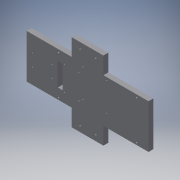
# Autodesk Inventor part: Основная пластина платформы
Saved by Autodesk Inventor 2019.1 (Build 231200000, 200)
## iProperties
Created: 2018-10-15
Part Number: Основная пластина платформы
Material: Типовые
Document SubType Name: Modeling
Designer: Олег
Density: 1 g/cm^3
Appearance: По умолчанию
Author: Олег
Autodesk Inventor part; units mm, degrees
ref_plane "YZ Plane" through (0, 0, 0) normal (1, 0, 0) x (0, 1, 0)
ref_plane "XZ Plane" through (0, 0, 0) normal (0, 1, 0) x (-1, 0, 0)
ref_plane "XY Plane" through (0, 0, 0) normal (0, 0, 1) x (1, 0, 0)
sketch "Эскиз1" plane through (0, 0, 0) normal (0, 0, 1) x (1, 0, 0)
  line L0 (-125, -45) -> (125, -45)
  line L1 (125, -45) -> (125, 45)
  line L2 (125, 45) -> (-125, 45)
  line L3 (-125, 45) -> (-125, -45)
  line L4 (-125, -45) -> (125, 45) construction
  line L5 (125, -45) -> (-125, 45) construction
  line L6 (32.5, -80) -> (-32.5, -80)
  line L7 (-32.5, -80) -> (-32.5, 80)
  line L8 (-32.5, 80) -> (32.5, 80)
  line L9 (32.5, 80) -> (32.5, -80)
  line L10 (32.5, -80) -> (-32.5, 80) construction
  line L11 (-32.5, -80) -> (32.5, 80) construction
  point P0 (0, 0)
  dimension "d0" = 250
  dimension "d1" = 90
  dimension "d2" = 65
  dimension "d3" = 160
  constraints: 24 end point, 4 midpoint, 4 parallel, 2 horizontal, 2 perpendicular
  measures "d0" distance of L2.end L1.end
  measures "d1" distance of L1.end L0.end
  measures "d2" distance of L7.end L8.end
  measures "d3" distance of L6.end L7.end
extrude "Выдавливание1" add sketch "Эскиз1" along normal blind 10
sketch "Эскиз2" plane through (0, 0, 10) normal (0, 0, 1) x (1, 0, 0)
  line L0 (16, 68) -> (-16, 68) construction
  line L1 (-16, 68) -> (-16, 80) construction
  line L2 (-16, 80) -> (16, 80) construction
  line L3 (16, 80) -> (16, 68) construction
  line L4 (16, 68) -> (-16, 80) construction
  line L5 (-16, 68) -> (16, 80) construction
  line L6 (0, 0) -> (16, 0) construction
  line L7 (16, -68) -> (-16, -68) construction
  line L8 (-16, -68) -> (-16, -80) construction
  line L9 (-16, -80) -> (16, -80) construction
  line L10 (16, -80) -> (16, -68) construction
  line L11 (16, -68) -> (-16, -80) construction
  line L12 (-16, -68) -> (16, -80) construction
  circle A0 centre (-16, 68) radius 2
  circle A1 centre (16, 68) radius 2
  circle A2 centre (-16, -68) radius 2
  circle A3 centre (16, -68) radius 2
  point P0 (0, 74)
  point P1 (-32.5, 80)
  point P2 (0, 74)
  point P3 (0, 74)
  point P4 (0, -74)
  point P5 (-32.5, -80)
  point P6 (0, -74)
  point P7 (0, -74)
  dimension "d6" = 32
  dimension "d7" = 12
  dimension "d8" = 4
  dimension "d9" = 4
  dimension "d10" = 4
  dimension "d11" = 4
  constraints: 26 end point, 8 symmetric about line, 6 midpoint, 4 centre point, 4 coincident, 2 horizontal, 2 parallel, 2 point on line, 1 perpendicular, 1 vertical alignment
  measures "d6" distance of L1.end L2.end
  measures "d7" distance of L0.end L1.end
  measures "d8" diameter of A0
  measures "d9" diameter of A1
  measures "d10" diameter of A2
  measures "d11" diameter of A3
extrude "Выдавливание2" cut sketch "Эскиз2" against normal blind 10
sketch "Эскиз3" plane through (0, 0, 10) normal (0, 0, 1) x (1, 0, 0)
  line L0 (100, -40) -> (-60, -40) construction
  line L1 (-60, -40) -> (-60, 40) construction
  line L2 (-60, 40) -> (100, 40) construction
  line L3 (100, 40) -> (100, -40) construction
  line L4 (100, -40) -> (-60, 40) construction
  line L5 (-60, -40) -> (100, 40) construction
  line L6 (125, -45) -> (125, 45) construction
  circle A0 centre (100, 40) radius 2
  circle A1 centre (100, -40) radius 2
  circle A2 centre (-60, -40) radius 2
  circle A3 centre (-60, 40) radius 2
  point P0 (0, 0)
  point P1 (20, 0)
  point P2 (20, 0)
  dimension "d14" = 160
  dimension "d15" = 80
  dimension "d16" = 25
  dimension "d17" = 4
  dimension "d18" = 4
  dimension "d19" = 4
  dimension "d20" = 4
  constraints: 12 end point, 4 centre point, 4 coincident, 3 midpoint, 2 parallel, 1 horizontal, 1 horizontal alignment, 1 perpendicular
  measures "d14" distance of L1.end L2.end
  measures "d15" distance of L0.end L1.end
  measures "d16" distance between parallel lines of L6 L3
  measures "d17" diameter of A0
  measures "d18" diameter of A1
  measures "d19" diameter of A2
  measures "d20" diameter of A3
extrude "Выдавливание3" cut sketch "Эскиз3" against normal blind 10
sketch "Эскиз4" plane through (0, 0, 10) normal (0, 0, 1) x (1, 0, 0)
  line L0 (-113, -12.5) -> (-73, -12.5) construction
  line L1 (-73, -12.5) -> (-73, 12.5) construction
  line L2 (-73, 12.5) -> (-113, 12.5) construction
  line L3 (-113, 12.5) -> (-113, -12.5) construction
  line L4 (-113, -12.5) -> (-73, 12.5) construction
  line L5 (-73, -12.5) -> (-113, 12.5) construction
  line L6 (-125, 45) -> (-125, -45) construction
  circle A0 centre (-113, 12.5) radius 1.5
  circle A1 centre (-73, 12.5) radius 1.5
  circle A2 centre (-73, -12.5) radius 1.5
  circle A3 centre (-113, -12.5) radius 1.5
  point P0 (0, 0)
  point P1 (-93, 0)
  point P2 (-93, 0)
  dimension "d23" = 40
  dimension "d24" = 25
  dimension "d25" = 12
  dimension "d26" = 3
  dimension "d27" = 3
  dimension "d28" = 3
  dimension "d29" = 3
  constraints: 12 end point, 4 centre point, 4 coincident, 3 midpoint, 2 parallel, 1 horizontal, 1 horizontal alignment, 1 perpendicular
  measures "d23" distance of L2.end L1.end
  measures "d24" distance of L1.end L0.end
  measures "d25" distance between parallel lines of L6 L3
  measures "d26" diameter of A0
  measures "d27" diameter of A1
  measures "d28" diameter of A2
  measures "d29" diameter of A3
extrude "Выдавливание4" cut sketch "Эскиз4" against normal blind 10
sketch "Эскиз5" plane through (0, 0, 10) normal (0, 0, 1) x (1, 0, 0)
  line L0 (-51, -23.5) -> (-61, -23.5)
  line L1 (-61, -23.5) -> (-61, 23.5)
  line L2 (-61, 23.5) -> (-51, 23.5)
  line L3 (-51, 23.5) -> (-51, -23.5)
  line L4 (-51, -23.5) -> (-61, 23.5) construction
  line L5 (-61, -23.5) -> (-51, 23.5) construction
  circle A0 centre (-73, 12.5) radius 1.5 projected
  point P0 (0, 0)
  point P1 (-56, 0)
  point P2 (-56, 0)
  dimension "d32" = 10
  dimension "d33" = 47
  dimension "d34" = 12
  constraints: 12 end point, 3 midpoint, 2 parallel, 1 horizontal, 1 horizontal alignment, 1 perpendicular
  measures "d32" distance of L1.end L2.end
  measures "d33" distance of L0.end L1.end
  measures "d34" distance from line of A0.centre L1
extrude "Выдавливание5" cut sketch "Эскиз5" against normal blind 10 contours L0 L1 L2 L3
sketch "Эскиз6" plane through (0, 0, 10) normal (0, 0, 1) x (1, 0, 0)
  line L0 (-18, -25) -> (-48, -25) construction
  line L1 (-48, -25) -> (-48, 25) construction
  line L2 (-48, 25) -> (-18, 25) construction
  line L3 (-18, 25) -> (-18, -25) construction
  line L4 (-18, -25) -> (-48, 25) construction
  line L5 (-48, -25) -> (-18, 25) construction
  line L6 (-51, 23.5) -> (-51, -23.5) construction
  circle A0 centre (-48, 25) radius 1.5
  circle A1 centre (-18, 25) radius 1.5
  circle A2 centre (-18, -25) radius 1.5
  circle A3 centre (-48, -25) radius 1.5
  point P0 (0, 0)
  point P1 (-33, 0)
  point P2 (-33, 0)
  dimension "d37" = 30
  dimension "d38" = 50
  dimension "d39" = 3
  dimension "d40" = 3
  dimension "d41" = 3
  dimension "d42" = 3
  dimension "d43" = 3
  constraints: 12 end point, 4 centre point, 4 coincident, 3 midpoint, 2 parallel, 1 horizontal, 1 horizontal alignment, 1 perpendicular
  measures "d37" distance of L1.end L2.end
  measures "d38" distance of L0.end L1.end
  measures "d39" distance between parallel lines of L6 L1
  measures "d40" diameter of A0
  measures "d41" diameter of A1
  measures "d42" diameter of A2
  measures "d43" diameter of A3
extrude "Выдавливание6" cut sketch "Эскиз6" against normal blind 10
sketch "Эскиз7" plane through (0, 0, 10) normal (0, 0, 1) x (1, 0, 0)
  circle A0 centre (-10, -18.5758) radius 1.375 projected
  circle A1 centre (39, -18.5758) radius 1.375 projected
  circle A2 centre (39, 39.4242) radius 1.375 projected
  circle A3 centre (-10, 39.4242) radius 1.375 projected
  point P0 (0, 0)
extrude "Выдавливание7" cut sketch "Эскиз7" against normal blind 10
